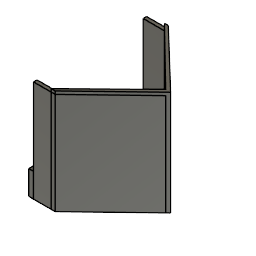
robotassem (Autodesk Fusion 360 archive; units mm, degrees)
design "robotpush"
Autodesk Fusion 360 part; units mm, degrees
sketch "Sketch1" plane through (0, 0, 0) normal (1, 0, 0) x (0, 1, 0)
  line L0 (-32.9565, 10.2616) -> (32.9565, 10.2616)
  line L1 (32.9565, 10.2616) -> (32.9565, 0)
  line L2 (32.9565, 0) -> (-32.9565, 0)
  line L3 (-32.9565, 0) -> (-32.9565, 10.2616)
  dimension "d2" = 65.913
  dimension "d3" = 10.2616
  constraint horizontal L0
  constraint vertical L1
  constraint horizontal L2
  constraint vertical L3
  constraint coincident origin L2
  constraint midpoint origin L2
  measures "d2" distance of L0.start L0.end
  measures "d3" distance of L0.end L1.end
extrude "Extrude1" add sketch "Sketch1" along normal blind 2 makes body 1
sketch "Sketch2" plane through (0, 0, 0) normal (0, 0, -1) x (1, 0, 0)
  line L0 (0, 32.9565) -> (0, -32.9565)
  line L1 (0, -32.9565) -> (2, -32.9565)
  line L2 (2, -32.9565) -> (2, 32.9565)
  line L3 (2, 32.9565) -> (0, 32.9565)
  line L4 (2, 32.9565) -> (36.29, 0)
  line L5 (2, 0) -> (36.29, 0) construction
  line L6 (2, -32.9565) -> (36.29, 0)
  line L7 (2, 32.9565) -> (2, 31.4565)
  line L8 (36.29, 0) -> (35.2085, -1.0394)
  line L9 (35.2085, -1.0394) -> (2, 31.4565)
  line L10 (35.2085, 1.0394) -> (2, -31.4565)
  line L11 (2, -32.9565) -> (2, -24.0665)
  line L12 (2, -24.0665) -> (11.2497, -24.0665)
  line L13 (2, -22.5665) -> (12.8104, -22.5665)
  line L14 (2, 24.0665) -> (11.2497, 24.0665)
  line L15 (2, 22.5665) -> (12.8104, 22.5665)
  dimension "d6" = 34.29
  dimension "d7" = 1.5
  dimension "d8" = 1.5
  dimension "d14" = 8.89
  dimension "d15" = 1.5
  constraint coincident L2.end L3.start
  constraint midpoint L2 L5.start
  constraint perpendicular L2 L5
  constraint coincident L4.end L5.end
  constraint symmetric L2.end L5 L1.end
  constraint symmetric L4.end L5 L6.end
  constraint coincident L2 L7.end
  constraint coincident L6 L8.end
  constraint symmetric L5 L7.end L10.end
  constraint symmetric L5 L8.end L10.start
  constraint coincident L1.end L2.start
  constraint coincident L2 L11.end
  constraint coincident L6 L12.end
  constraint perpendicular L11 L12
  constraint coincident L2 L13.start
  constraint coincident L6 L13.end
  constraint perpendicular L2 L13
  constraint symmetric L5 L11.end L14.start
  constraint symmetric L5 L12.end L14.end
  constraint symmetric L5 L13.start L15.start
  constraint symmetric L5 L13.end L15.end
  measures "d6" distance of L5.start L4.end
  measures "d7" distance of L2.end L7.end
  measures "d8" distance of L4.end L8.end
  measures "d14" distance of L1.end L11.end
  measures "d15" distance of L11.end L13.start
extrude "Extrude2" add sketch "Sketch2" against normal blind 44.45 contours L2 L4 L7 L9 L14 | L2 L6 L10 L11 L12 | L4 L9 L14 L15 | L6 L10 L12 L13 | L4 L9 L10 L15 | L6 L9 L10 L13 | L4 L6 L8 L9 L10 bodies 1
sketch "Sketch3" plane through (0, 0, 0) normal (-1, 0, 0) x (0, -1, 0)
  line L0 (-32.9565, 0) -> (32.9565, 0)
  line L1 (32.9565, 0) -> (32.9565, 10.2616)
  line L2 (32.9565, 10.2616) -> (-32.9565, 10.2616)
  line L3 (-32.9565, 10.2616) -> (-32.9565, 0)
  line L4 (32.9565, 0) -> (-32.9565, 10.2616) construction
  line L5 (32.9565, 10.2616) -> (-32.9565, 0) construction
  line L6 (32.9565, 0) -> (0, 10.2616) construction
  line L7 (32.9565, 10.2616) -> (0, 0) construction
  line L8 (0, 5.1308) -> (0, -10.6612) construction
  circle A0 centre (16.4782, 5.1308) radius 1.524
  circle A1 centre (-16.4782, 5.1308) radius 1.524
  dimension "d11" = 3.048
  constraint coincident L0.end L1.start
  constraint coincident L2.end L3.start
  constraint coincident L1.end L2.start
  constraint coincident L0.start L3.end
  constraint midpoint L2 L6.end
  constraint coincident L7.end origin
  constraint midpoint L4 L8.start
  constraint vertical L8
  constraint midpoint L6 A0.centre
  constraint symmetric L8 A0 A1
  measures "d11" diameter of A0
extrude "Extrude3" cut sketch "Sketch3" against normal blind 7 contours A0 | A1 bodies 1
extrude "Extrude4" add sketch "Sketch2" against normal blind 43.18 separate body contours L4 L9 L14 L15 | L6 L10 L12 L13 | L2 L9 L14 L15 | L4 L9 L10 L15 | L2 L10 L12 L13 | L6 L9 L10 L13 makes body 2
sketch "Sketch4" plane through (0, 0, 0) normal (0, 0, -1) x (1, 0, 0)
sketch "Sketch5" plane through (0, 0, 0) normal (0, 0, -1) x (1, 0, 0)
  line L0 (18.1994, -36.4141) -> (-7.2179, -36.4141)
  line L1 (-7.2179, -36.4141) -> (-7.2179, -24.0665)
  line L2 (-7.2179, -24.0665) -> (18.1994, -24.0665)
  line L3 (18.1994, -24.0665) -> (18.1994, -36.4141)
  line L4 (28.1513, -24.0665) -> (2, -24.0665)
  line L5 (0, 0) -> (47.1507, 0) construction
  line L6 (18.1994, 36.4141) -> (-7.2179, 36.4141)
  line L7 (18.1994, 24.0665) -> (18.1994, 36.4141)
  line L8 (-7.2179, 36.4141) -> (-7.2179, 24.0665)
  line L9 (-7.2179, 24.0665) -> (18.1994, 24.0665)
  point P0 (2, -24.0665)
  dimension "d18" = 25.4173
  dimension "d19" = 12.3476
  constraint horizontal L0
  constraint vertical L1
  constraint horizontal L2
  constraint vertical L3
  constraint parallel L2 L4
  constraint coincident P0 L4.end
  constraint coincident L2 P0
  constraint coincident L5.start origin
  constraint horizontal L5
  constraint symmetric L0.start L5 L6.start
  constraint symmetric L0.end L5 L6.end
  constraint symmetric L1.end L5 L8.end
  constraint symmetric L2.end L5 L7.start
  measures "d18" distance of L0.start L0.end
  measures "d19" distance of L0.end L1.end
extrude "Extrude5" cut sketch "Sketch5" against normal blind 51 bodies 1 makes body 3 at (19.5965, 16.0443, 14.8167)
